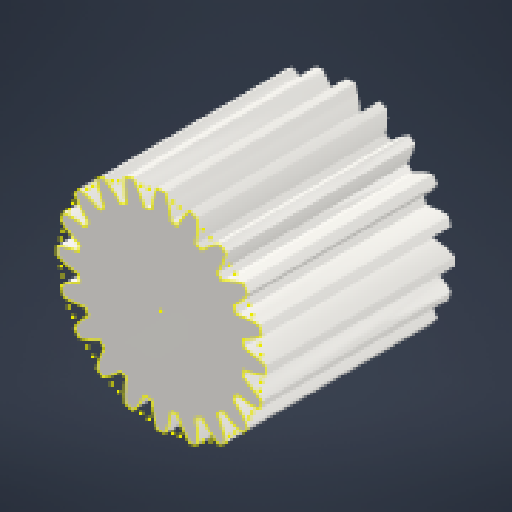
# Autodesk Inventor part: Цилиндрическое зубчатое зацепление1
Saved by Autodesk Inventor 2025 (Build 290162000, 162)
## iProperties
CustomPartVersion: 1
Created: 2025-01-15
Part Number: Цилиндрическое зубчатое зацепление1
Material: Steel
Document SubType Name: Modeling
Designer: Phantom
Categories: <?xml version="1.0" encoding="UTF-16"?> <MemberInstance><Categories><FamilyTemplate><FamilyTemplateParameter ValueType="xs:double" Id="1" ObjectReferenceKey="da_z" ObjectType="kUserParameterObject"/><FamilyTemplateParameter ValueType="xs:double" Id="2" ObjectReferenceKey="da_b" ObjectType="kUserParameterObject"/><FamilyTemplateParameter ValueType="xs:double" Id="3" ObjectReferenceKey="da_beta" ObjectType="kUserParameterObject"/><FamilyTemplateParameter ValueType="xs:double" Id="4" ObjectReferenceKey="da_da" ObjectType="kUserParameterObject"/><FamilyTemplateParameter ValueType="xs:double" Id="5" ObjectReferenceKey="da_aw" ObjectType="kUserParameterObject"/><FamilyTemplateParameter ValueType="xs:string" Id="6" ObjectReferenceKey="EAIAABAAAACIAQAAAAAAAIAAAAAAAAAA" ObjectType="83910656" SubObjectId="SurfaceGeometry"/></FamilyTemplate><ParamToTemplateMap><ParamToTemplate CategoryParameter="//CategoryParameter[@InternalName='046C89C9-8512-4d59-83FE-43B91F4F132A']" TemplateParameter="1"/><ParamToTemplate CategoryParameter="//CategoryParameter[@InternalName='2552DF32-E462-4b46-AEBF-C6C7768E72AC']" TemplateParameter="2"/><ParamToTemplate CategoryParameter="//CategoryParameter[@InternalName='C9EE641D-15FC-4fae-A226-E94C4372FDD7']" TemplateParameter="3"/><ParamToTemplate><ParamToTemplate CategoryParameter="//CategoryParameter[@InternalName='00B6519A-459B-49c7-AD84-2E56D39A5744']" ConstantValue="0.000000"/></ParamToTemplate><ParamToTemplate><ParamToTemplate CategoryParameter="//CategoryParameter[@InternalName='04B31F0E-C7A6-4894-AA32-9629BEFACF47']" ConstantValue="1.000000"/></ParamToTemplate><ParamToTemplate><ParamToTemplate CategoryParameter="//CategoryParameter[@InternalName='43CBEC2E-7847-49e7-A936-2F7889FCB2D9']" ConstantValue="0.250000"/></ParamToTemplate><ParamToTemplate><ParamToTemplate CategoryParameter="//CategoryParameter[@InternalName='B1EFC894-105D-4ebd-86BF-FA20ED196853']" ConstantValue="0.350000"/></ParamToTemplate><ParamToTemplate><ParamToTemplate CategoryParameter="//CategoryParameter[@InternalName='51175063-3D10-4879-93E8-6246FE8B403D']" ConstantValue="2060000000.000000"/></ParamToTemplate><ParamToTemplate><ParamToTemplate CategoryParameter="//CategoryParameter[@InternalName='A3A52E27-4454-46a9-B0BD-C932399B70AF']" ConstantValue="0.300000"/></ParamToTemplate><ParamToTemplate><ParamToTemplate CategoryParameter="//CategoryParameter[@InternalName='91B76062-C214-41d9-B1B9-14D2AB99603D']" ConstantValue="0.100000"/></ParamToTemplate><ParamToTemplate><ParamToTemplate CategoryParameter="//CategoryParameter[@InternalName='374E806E-8B8A-4dda-A9AA-1039D6500AD2']" ConstantValue="10.000000"/></ParamToTemplate><ParamToTemplate><ParamToTemplate CategoryParameter="//CategoryParameter[@InternalName='2D373A89-B862-43d6-8D0B-0CBF12AB9F6C']" ConstantValue="0.349066"/></ParamToTemplate><ParamToTemplate CategoryParameter="//CategoryParameter[@InternalName='37777632-D6A2-4fac-9D53-DB8ACD95C989']" TemplateParameter="4"/><ParamToTemplate CategoryParameter="//CategoryParameter[@InternalName='FD1017F1-B727-4f7e-9707-0F86F1FF9423']" TemplateParameter="5"/><ParamToTemplate><ParamToTemplate CategoryParameter="//CategoryParameter[@InternalName='9E1B4470-B2D3-4ff1-B813-535BB4CDF51A']" ConstantValue="3520000.000000"/></ParamToTemplate><ParamToTemplate><ParamToTemplate CategoryParameter="//CategoryParameter[@InternalName='F8452263-BFF6-458c-9FB1-07C4B99E95CD']" ConstantValue="11400000.000000"/></ParamToTemplate><ParamToTemplate><ParamToTemplate CategoryParameter="//CategoryParameter[@InternalName='3E3BB259-FD49-497f-8171-6EBC954A3479']" ConstantValue="2.000000"/></ParamToTemplate><ParamToTemplate CategoryParameter="//CategoryParameter[@InternalName='27C3BAF2-7550-4e4b-AE2C-0DB134B7D9B7']" TemplateParameter="6"/></ParamToTemplateMap><Category DisplayName="Gear" InternalName="DC85795E-93AB-48d5-8EEE-5A27447B64BD" Mnemonic="Gear"><CategoryParameter DisplayName="z" InternalName="046C89C9-8512-4d59-83FE-43B91F4F132A" Mnemonic="z"/><CategoryParameter DisplayName="b" InternalName="2552DF32-E462-4b46-AEBF-C6C7768E72AC" Mnemonic="b"/><CategoryParameter DisplayName="||b|" InternalName="C9EE641D-15FC-4fae-A226-E94C4372FDD7" Mnemonic="beta"/><CategoryParameter DisplayName="x" InternalName="00B6519A-459B-49c7-AD84-2E56D39A5744" Mnemonic="x"/><CategoryParameter DisplayName="a*" InternalName="04B31F0E-C7A6-4894-AA32-9629BEFACF47" Mnemonic="a"/><CategoryParameter DisplayName="c*" InternalName="43CBEC2E-7847-49e7-A936-2F7889FCB2D9" Mnemonic="c"/><CategoryParameter DisplayName="r|.f|*" InternalName="B1EFC894-105D-4ebd-86BF-FA20ED196853" Mnemonic="rf"/><CategoryParameter DisplayName="E" InternalName="51175063-3D10-4879-93E8-6246FE8B403D" Mnemonic="E"/><CategoryParameter DisplayName="||m|" InternalName="A3A52E27-4454-46a9-B0BD-C932399B70AF" Mnemonic="mi"/><Category DisplayName="SpurGear" InternalName="26C5A22E-A91E-4dfd-A3B3-23CCAFAE1764" Mnemonic="SpurGear"><CategoryParameter DisplayName="m" InternalName="91B76062-C214-41d9-B1B9-14D2AB99603D" Mnemonic="m"/><CategoryParameter DisplayName="P" InternalName="374E806E-8B8A-4dda-A9AA-1039D6500AD2" Mnemonic="PP"/><CategoryParameter DisplayName="||a|" InternalName="2D373A89-B862-43d6-8D0B-0CBF12AB9F6C" Mnemonic="alpha"/><CategoryParameter DisplayName="d|.a|" InternalName="37777632-D6A2-4fac-9D53-DB8ACD95C989" Mnemonic="da"/><CategoryParameter DisplayName="a|.w|" InternalName="FD1017F1-B727-4f7e-9707-0F86F1FF9423" Mnemonic="aw"/><CategoryParameter DisplayName="||s||.Flim|" InternalName="9E1B4470-B2D3-4ff1-B813-535BB4CDF51A" Mnemonic="sFlim"/><CategoryParameter DisplayName="||s||.Hlim|" InternalName="F8452263-BFF6-458c-9FB1-07C4B99E95CD" Mnemonic="sHlim"/><CategoryParameter DisplayName="тип" InternalName="3E3BB259-FD49-497f-8171-6EBC954A3479" Mnemonic="type"/><CategoryParameter DisplayName="PitchDiameter" InternalName="27C3BAF2-7550-4e4b-AE2C-0DB134B7D9B7" Mnemonic="IDS_PITCHDIAM"/></Category></Category></Categories></MemberInstance>
Density: 1 g/cm^3
Appearance: Steel
Author: Phantom
Autodesk Inventor part; units mm, degrees
sketch "Sketch1" plane through (0, 0, 0) normal (0, 0, 1) x (1, 0, 0)
  circle A0 centre (0, 0) radius 11
  dimension "d0" = 22
  constraints: 1 centre point
  measures "d0" diameter of A0
extrude "Extrusion1" add sketch "Sketch1" along normal blind 20
ref_plane "Work Plane2" through (0, 0, 10) normal (0, 0, 1) x (1, 0, 0)
sketch "Sketch2" plane through (0, 0, 0) normal (0, 0, -1) x (-1, 0, 0)
  circle A0 centre (0, 0) radius 11 projected
  circle A1 centre (0, 0) radius 10
  dimension "d3" = 20
  constraints: 1 centre point, 1 coincident
  measures "d3" diameter of A1
surface extrude "Средний диаметр" sketch "Sketch2" against normal through all shown no curves A1
ref_plane "Work Plane8" through (0, 0, 0) normal (0.9876883, 0.1564345, 0) x (0, 0, 1)
ref_plane "Work Plane9" through (0, 0, 0) normal (1, 0, 0) x (0, 1, 0)
spur gear teeth "Цилиндрическое зубчатое зацепление" teeth 20 pitch diameter 20 tip diameter 22 root diameter 17.5 face width 20 start plane through (0, 0, 0) normal (0, 0, -1) x (-1, 0, 0)
sketch "Эскиз3" plane through (0, 0, 20) normal (0, 0, 1) x (1, 0, 0)
  arc A0 (-2.9858, 10.587) -> (-3.8073, 10.3201) centre (0, 0) ccw projected
  arc A1 (-3.8073, 10.3201) -> (-3.6633, 7.9463) centre (4.4532, 9.6299) ccw projected
  arc A2 (-3.6633, 7.9463) -> (-4.2754, 7.6343) centre (0, 0) ccw projected
  arc A3 (-4.2754, 7.6343) -> (-6.1113, 9.1462) centre (-10.4083, 2.0576) ccw projected
  arc A4 (-6.1113, 9.1462) -> (-6.81, 8.6385) centre (0, 0) ccw projected
  arc A5 (-6.81, 8.6385) -> (-5.9395, 6.4253) centre (1.2594, 10.5347) ccw projected
  arc A6 (-5.9395, 6.4253) -> (-6.4253, 5.9395) centre (0, 0) ccw projected
  arc A7 (-6.4253, 5.9395) -> (-8.6385, 6.81) centre (-10.5347, -1.2594) ccw projected
  arc A8 (-8.6385, 6.81) -> (-9.1462, 6.1113) centre (0, 0) ccw projected
  arc A9 (-9.1462, 6.1113) -> (-7.6343, 4.2754) centre (-2.0576, 10.4083) ccw projected
  arc A10 (-7.6343, 4.2754) -> (-7.9463, 3.6633) centre (0, 0) ccw projected
  arc A11 (-7.9463, 3.6633) -> (-10.3201, 3.8073) centre (-9.6299, -4.4532) ccw projected
  arc A12 (-10.3201, 3.8073) -> (-10.587, 2.9858) centre (0, 0) ccw projected
  arc A13 (-10.587, 2.9858) -> (-8.5819, 1.707) centre (-5.1733, 9.263) ccw projected
  arc A14 (-8.5819, 1.707) -> (-8.6893, 1.0285) centre (0, 0) ccw projected
  arc A15 (-8.6893, 1.0285) -> (-10.9915, 0.4319) centre (-7.7825, -7.211) ccw projected
  arc A16 (-10.9915, 0.4319) -> (-10.9915, -0.4319) centre (0, 0) ccw projected
  arc A17 (-10.9915, -0.4319) -> (-8.6893, -1.0285) centre (-7.7825, 7.211) ccw projected
  arc A18 (-8.6893, -1.0285) -> (-8.5819, -1.707) centre (0, 0) ccw projected
  arc A19 (-8.5819, -1.707) -> (-10.587, -2.9858) centre (-5.1733, -9.263) ccw projected
  arc A20 (-10.587, -2.9858) -> (-10.3201, -3.8073) centre (0, 0) ccw projected
  arc A21 (-10.3201, -3.8073) -> (-7.9463, -3.6633) centre (-9.6299, 4.4532) ccw projected
  arc A22 (-7.9463, -3.6633) -> (-7.6343, -4.2754) centre (0, 0) ccw projected
  arc A23 (-7.6343, -4.2754) -> (-9.1462, -6.1113) centre (-2.0576, -10.4083) ccw projected
  arc A24 (-9.1462, -6.1113) -> (-8.6385, -6.81) centre (0, 0) ccw projected
  arc A25 (-8.6385, -6.81) -> (-6.4253, -5.9395) centre (-10.5347, 1.2594) ccw projected
  arc A26 (-6.4253, -5.9395) -> (-5.9395, -6.4253) centre (0, 0) ccw projected
  arc A27 (-5.9395, -6.4253) -> (-6.81, -8.6385) centre (1.2594, -10.5347) ccw projected
  arc A28 (-6.81, -8.6385) -> (-6.1113, -9.1462) centre (0, 0) ccw projected
  arc A29 (-6.1113, -9.1462) -> (-4.2754, -7.6343) centre (-10.4083, -2.0576) ccw projected
  arc A30 (-4.2754, -7.6343) -> (-3.6633, -7.9463) centre (0, 0) ccw projected
  arc A31 (-3.6633, -7.9463) -> (-3.8073, -10.3201) centre (4.4532, -9.6299) ccw projected
  arc A32 (-3.8073, -10.3201) -> (-2.9858, -10.587) centre (0, 0) ccw projected
  arc A33 (-2.9858, -10.587) -> (-1.707, -8.5819) centre (-9.263, -5.1733) ccw projected
  arc A34 (-1.707, -8.5819) -> (-1.0285, -8.6893) centre (0, 0) ccw projected
  arc A35 (-1.0285, -8.6893) -> (-0.4319, -10.9915) centre (7.211, -7.7825) ccw projected
  arc A36 (-0.4319, -10.9915) -> (0.4319, -10.9915) centre (0, 0) ccw projected
  arc A37 (0.4319, -10.9915) -> (1.0285, -8.6893) centre (-7.211, -7.7825) ccw projected
  arc A38 (1.0285, -8.6893) -> (1.707, -8.5819) centre (0, 0) ccw projected
  arc A39 (1.707, -8.5819) -> (2.9858, -10.587) centre (9.263, -5.1733) ccw projected
  arc A40 (2.9858, -10.587) -> (3.8073, -10.3201) centre (0, 0) ccw projected
  arc A41 (3.8073, -10.3201) -> (3.6633, -7.9463) centre (-4.4532, -9.6299) ccw projected
  arc A42 (3.6633, -7.9463) -> (4.2754, -7.6343) centre (0, 0) ccw projected
  arc A43 (4.2754, -7.6343) -> (6.1113, -9.1462) centre (10.4083, -2.0576) ccw projected
  arc A44 (6.1113, -9.1462) -> (6.81, -8.6385) centre (0, 0) ccw projected
  arc A45 (6.81, -8.6385) -> (5.9395, -6.4253) centre (-1.2594, -10.5347) ccw projected
  arc A46 (5.9395, -6.4253) -> (6.4253, -5.9395) centre (0, 0) ccw projected
  arc A47 (6.4253, -5.9395) -> (8.6385, -6.81) centre (10.5347, 1.2594) ccw projected
  arc A48 (8.6385, -6.81) -> (9.1462, -6.1113) centre (0, 0) ccw projected
  arc A49 (9.1462, -6.1113) -> (7.6343, -4.2754) centre (2.0576, -10.4083) ccw projected
  arc A50 (7.6343, -4.2754) -> (7.9463, -3.6633) centre (0, 0) ccw projected
  arc A51 (7.9463, -3.6633) -> (10.3201, -3.8073) centre (9.6299, 4.4532) ccw projected
  arc A52 (10.3201, -3.8073) -> (10.587, -2.9858) centre (0, 0) ccw projected
  arc A53 (10.587, -2.9858) -> (8.5819, -1.707) centre (5.1733, -9.263) ccw projected
  arc A54 (8.5819, -1.707) -> (8.6893, -1.0285) centre (0, 0) ccw projected
  arc A55 (8.6893, -1.0285) -> (10.9915, -0.4319) centre (7.7825, 7.211) ccw projected
  arc A56 (10.9915, -0.4319) -> (10.9915, 0.4319) centre (0, 0) ccw projected
  arc A57 (10.9915, 0.4319) -> (8.6893, 1.0285) centre (7.7825, -7.211) ccw projected
  arc A58 (8.6893, 1.0285) -> (8.5819, 1.707) centre (0, 0) ccw projected
  arc A59 (8.5819, 1.707) -> (10.587, 2.9858) centre (5.1733, 9.263) ccw projected
  arc A60 (10.587, 2.9858) -> (10.3201, 3.8073) centre (0, 0) ccw projected
  arc A61 (10.3201, 3.8073) -> (7.9463, 3.6633) centre (9.6299, -4.4532) ccw projected
  arc A62 (7.9463, 3.6633) -> (7.6343, 4.2754) centre (0, 0) ccw projected
  arc A63 (7.6343, 4.2754) -> (9.1462, 6.1113) centre (2.0576, 10.4083) ccw projected
  arc A64 (9.1462, 6.1113) -> (8.6385, 6.81) centre (0, 0) ccw projected
  arc A65 (8.6385, 6.81) -> (6.4253, 5.9395) centre (10.5347, -1.2594) ccw projected
  arc A66 (6.4253, 5.9395) -> (5.9395, 6.4253) centre (0, 0) ccw projected
  arc A67 (5.9395, 6.4253) -> (6.81, 8.6385) centre (-1.2594, 10.5347) ccw projected
  arc A68 (6.81, 8.6385) -> (6.1113, 9.1462) centre (0, 0) ccw projected
  arc A69 (6.1113, 9.1462) -> (4.2754, 7.6343) centre (10.4083, 2.0576) ccw projected
  arc A70 (4.2754, 7.6343) -> (3.6633, 7.9463) centre (0, 0) ccw projected
  arc A71 (3.6633, 7.9463) -> (3.8073, 10.3201) centre (-4.4532, 9.6299) ccw projected
  arc A72 (3.8073, 10.3201) -> (2.9858, 10.587) centre (0, 0) ccw projected
  arc A73 (2.9858, 10.587) -> (1.707, 8.5819) centre (9.263, 5.1733) ccw projected
  arc A74 (1.707, 8.5819) -> (1.0285, 8.6893) centre (0, 0) ccw projected
  arc A75 (1.0285, 8.6893) -> (0.4319, 10.9915) centre (-7.211, 7.7825) ccw projected
  arc A76 (0.4319, 10.9915) -> (-0.4319, 10.9915) centre (0, 0) ccw projected
  arc A77 (-0.4319, 10.9915) -> (-1.0285, 8.6893) centre (7.211, 7.7825) ccw projected
  arc A78 (-1.0285, 8.6893) -> (-1.707, 8.5819) centre (0, 0) ccw projected
  arc A79 (-1.707, 8.5819) -> (-2.9858, 10.587) centre (-9.263, 5.1733) ccw projected
equation "\"d0\" = da_da"
equation "\"d1\" = da_b"
equation "\"d3\" = da_d"
equation "\"d16\" = da_aw"
equation "\"d43\" = da_aw"
equation "\"d46\" = da_aw"
equation "\"da_da\" = 22"
equation "\"da_b\" = 20"
equation "\"da_d\" = 20"
equation "\"da_aw\" = 24"
body "Solid1"
body "Srf1"
